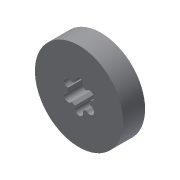
# Autodesk Inventor part: augmented gear v2
Saved by Autodesk Inventor 2014 (Build 180170000, 170)
## iProperties
Created: 2014-02-23
Part Number: augmented gear v2
Material: Generic
Document SubType Name: Modeling
Designer: Owner
Density: 1 g/cm^3
Appearance: Default
Author: Owner
Autodesk Inventor part; units mm, degrees
ref_plane "YZ Plane" through (0, 0, 0) normal (1, 0, 0) x (0, 1, 0)
ref_plane "XZ Plane" through (0, 0, 0) normal (0, 1, 0) x (-1, 0, 0)
ref_plane "XY Plane" through (0, 0, 0) normal (0, 0, 1) x (1, 0, 0)
sketch "Sketch1" plane through (0, 0, 0) normal (0, 0, 1) x (1, 0, 0)
  line L0 (7.8314, 13.1968) -> (7.8314, 20.4485) construction
  line L1 (7.8314, 13.1968) -> (14.1116, 16.8227) construction
  circle A0 centre (7.8314, 13.1968) radius 6.35 construction
  line L2 (7.8314, 13.1968) -> (14.1116, 9.571) construction
  line L3 (7.8314, 13.1968) -> (7.8314, 5.9451) construction
  line L4 (7.8314, 13.1968) -> (1.5513, 9.571) construction
  line L5 (7.8314, 13.1968) -> (1.5513, 16.8227) construction
  line L6 (7.8314, 20.4485) -> (14.1116, 16.8227)
  line L7 (14.1116, 16.8227) -> (14.1116, 9.571)
  line L8 (7.8314, 5.9451) -> (14.1116, 9.571)
  line L9 (7.8314, 5.9451) -> (1.5513, 9.571)
  line L10 (1.5513, 9.571) -> (1.5513, 16.8227)
  line L11 (1.5513, 16.8227) -> (7.8314, 20.4485)
  circle A1 centre (7.8314, 13.1968) radius 25.4
  circle A2 centre (7.8314, 20.4485) radius 2.3813
  circle A3 centre (14.1116, 16.8227) radius 2.3813
  circle A4 centre (14.1116, 9.571) radius 2.3813
  circle A5 centre (7.8314, 5.9451) radius 2.3813
  circle A6 centre (1.5513, 9.571) radius 2.3813
  circle A7 centre (1.5513, 16.8227) radius 2.3813
  line L12 (5.4502, 19.9903) -> (10.2127, 19.9903)
  line L13 (10.2127, 19.9903) -> (10.2127, 19.0737)
  line L14 (10.2127, 19.0737) -> (5.4502, 19.0737)
  line L15 (5.4502, 19.0737) -> (5.4502, 19.9903)
  line L16 (11.9019, 8.2952) -> (12.6147, 7.719)
  line L17 (12.6147, 7.719) -> (15.6085, 11.4229)
  line L18 (15.6085, 11.4229) -> (14.8957, 11.9991)
  line L19 (14.8957, 11.9991) -> (11.9019, 8.2952)
  line L20 (5.4502, 7.3199) -> (5.4502, 6.4034)
  line L21 (5.4502, 6.4034) -> (10.2127, 6.4034)
  line L22 (10.2127, 6.4034) -> (10.2127, 7.3199)
  line L23 (10.2127, 7.3199) -> (5.4502, 7.3199)
  line L24 (1.5513, 12.1225) -> (0.6959, 11.7933)
  line L25 (0.6959, 11.7933) -> (2.4066, 7.3487)
  line L26 (2.4066, 7.3487) -> (3.262, 7.6779)
  line L27 (3.262, 7.6779) -> (1.5513, 12.1225)
  line L28 (3.761, 18.0984) -> (3.0482, 18.6746)
  line L29 (3.0482, 18.6746) -> (0.0544, 14.9707)
  line L30 (0.0544, 14.9707) -> (0.7672, 14.3946)
  line L31 (0.7672, 14.3946) -> (3.761, 18.0984)
  line L32 (14.1116, 14.073) -> (14.9053, 14.5313)
  line L33 (14.9053, 14.5313) -> (12.5241, 18.6558)
  line L34 (12.5241, 18.6558) -> (11.7303, 18.1975)
  line L35 (11.7303, 18.1975) -> (14.1116, 14.073)
  circle A8 centre (7.8314, 13.1968) radius 4.0132 construction
  dimension "d9" = 4.7625
  dimension "d11" = 4.7625
  dimension "d0" = 7.2517
  dimension "d1" = 12.7
  dimension "d2" = 60
  dimension "d3" = 60
  dimension "d4" = 60
  dimension "d5" = 60
  dimension "d6" = 60
  dimension "d7" = 4.7625
  dimension "d8" = 4.7625
  dimension "d10" = 4.7625
  dimension "d12" = 4.7625
  dimension "d13" = 50.8
  dimension "d14" = 0.9165
  dimension "d16" = 0.9165
  dimension "d17" = 0.9165
  dimension "d18" = 0.9165
  dimension "d19" = 0.9165
  dimension "d20" = 0.9165
  dimension "d24" = 2.3368
  constraints: 72 end point, 14 parallel, 9 coincident, 8 tangent, 7 centre point, 7 point on line, 6 perpendicular, 5 equal length, 2 horizontal, 1 vertical, 10 other
  measures "d0" distance of L0.start L0.end
  measures "d1" diameter of A0
  measures "d2" angle of L1 L0
  measures "d3" angle of L2 L1
  measures "d4" angle of L3 L2
  measures "d5" angle of L4 L3
  measures "d6" angle of L5 L4
  measures "d7" diameter of A2
  measures "d8" diameter of A3
  measures "d10" diameter of A5
  measures "d12" diameter of A7
  measures "d13" diameter of A1
  measures "d14" distance of L12.end L13.end
  measures "d16" distance of L16.start L16.end
  measures "d17" distance of L20.start L20.end
  measures "d18" distance of L25.end L26.end
  measures "d19" distance of L28.start L28.end
  measures "d20" distance of L32.start L32.end
  measures "d24" radial gap between concentric circles of A8 A0
extrude "Extrusion1" add sketch "Sketch1" against normal blind 12.7
equation "\"d9\" = d7"
equation "\"d11\" = d7"
equation "\"d8\" = d7"
equation "\"d10\" = d7"
equation "\"d12\" = d7"
body "Solid1"
